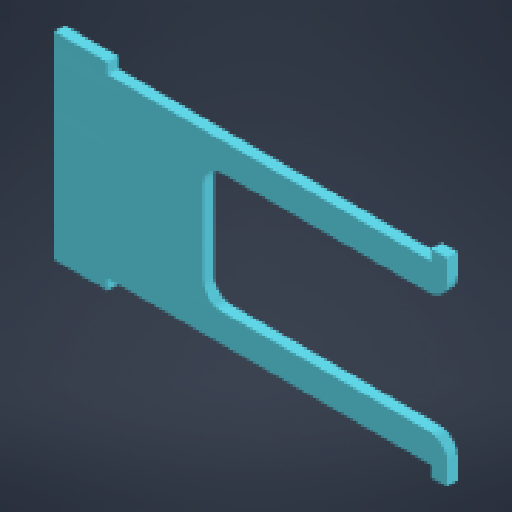
# Autodesk Inventor part: femur_reinforcement_tibea_steel
Saved by Autodesk Inventor 2026 (Build 300175000, 175)
## iProperties
Created: 2026-05-03
Part Number: femur_reinforcement_tibea_steel
Material: Сталь
Document SubType Name: Modeling
Designer: user
Density: 7.85 g/cm^3
Appearance: Серо-синий
Author: user
Autodesk Inventor part; units mm, degrees
ref_plane "YZ Plane" through (0, 0, 0) normal (1, 0, 0) x (0, 1, 0)
ref_plane "XZ Plane" through (0, 0, 0) normal (0, 1, 0) x (-1, 0, 0)
ref_plane "XY Plane" through (0, 0, 0) normal (0, 0, 1) x (1, 0, 0)
sketch "Эскиз3" plane through (0, 0, 0) normal (0, 0, 1) x (1, 0, 0)
  line L0 (106.2, 49.8) -> (15, 49.8)
  line L1 (0, 49.8) -> (0, 0)
  line L2 (0, 0) -> (0, -3)
  line L3 (0, -3) -> (15, -3)
  line L4 (15, -3) -> (15, 0)
  line L5 (0, 49.8) -> (0, 52.8)
  line L6 (0, 52.8) -> (15, 52.8)
  line L7 (15, 52.8) -> (15, 49.8)
  line L8 (138.7, 5.7) -> (47, 5.7)
  line L9 (42, 10.7) -> (42, 39.1)
  line L10 (47, 44.1) -> (105.7, 44.1)
  line L11 (110.7, 49.1) -> (110.7, 52.8)
  line L12 (110.7, 52.8) -> (106.2, 52.8)
  line L13 (106.2, 52.8) -> (106.2, 49.8)
  arc A0 (105.7, 44.1) -> (110.7, 49.1) centre (105.7, 49.1) ccw
  arc A1 (42, 10.7) -> (47, 5.7) centre (47, 10.7) ccw
  arc A2 (47, 44.1) -> (42, 39.1) centre (47, 39.1) ccw
  line L14 (15, 0) -> (139.2, 0)
  line L15 (139.2, 0) -> (139.2, -3)
  line L16 (139.2, -3) -> (143.7, -3)
  line L17 (143.7, -3) -> (143.7, 0.7)
  arc A3 (143.7, 0.7) -> (138.7, 5.7) centre (138.7, 0.7) ccw
  point P0 (42, 5.7)
  point P1 (42, 44.1)
  point P2 (110.7, 44.1)
  point P3 (143.7, 5.7)
  dimension "d10" = 15
  dimension "d12" = 42
  dimension "d13" = 4.5
  dimension "d14" = 5
  dimension "d15" = 5.7
  dimension "d16" = 5
  dimension "d17" = 91.2
  dimension "d18" = 3
  dimension "d20" = 5
  dimension "d21" = 124.2
  dimension "d22" = 49.8
  constraints: 36 end point, 9 perpendicular, 9 point on line, 8 point on circle, 8 tangent, 5 equal length, 4 centre point, 3 vertical, 2 horizontal, 1 equal radius, 1 vertical alignment, 1 other
  measures "d10" distance between parallel lines of L2 L4
  measures "d12" distance between parallel lines of L1 L9
  measures "d13" distance between parallel lines of L11 L13
  measures "d14" radius of A0
  measures "d15" distance between parallel lines of L10 L0
  measures "d16" radius of A1
  measures "d17" distance of L0.start L0.end
  measures "d18" distance of L3.end L4.end
  measures "d20" radius of A3
  measures "d21" distance between parallel lines of L4 L15
  measures "d22" distance between parallel lines of L0 L14
extrude "Выдавливание3" add sketch "Эскиз3" along normal blind 3
equation "\"d6\" = thickness_steel"
equation "\"tolerance_plazma\" = 0.1"
equation "\"thickness_steel\" = 3"
equation "\"d_main_screw_holes\" = 6.1"
equation "\"thickness_profile_tibea\" = 3"
equation "\"hight_shaft_shift\" = 37"
equation "\"thickness_profile_femur\" = 3"
equation "\"width_shaft_shift\" = 35"
equation "\"width_flattened_surface\" = 12"
